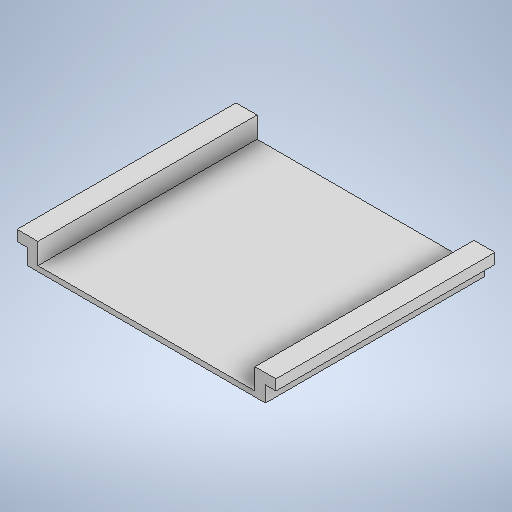
# Autodesk Inventor part: Avionics Cradle (12-13)
Saved by Autodesk Inventor 2025.2 (Build 292293000, 293)
## iProperties
Created: 2025-01-28
Part Number: Avionics Cradle (12-13)
Material: Generic
Document SubType Name: Modeling
Designer: Tia
Density: 1 g/cm^3
Appearance: Default
Author: Tia
Autodesk Inventor part; units mm, degrees
ref_plane "YZ Plane" through (0, 0, 0) normal (1, 0, 0) x (0, 1, 0)
ref_plane "XZ Plane" through (0, 0, 0) normal (0, 1, 0) x (-1, 0, 0)
ref_plane "XY Plane" through (0, 0, 0) normal (0, 0, 1) x (1, 0, 0)
sketch "Sketch2" plane through (0, 0, 0) normal (0, 0, 1) x (1, 0, 0)
  line L0 (-14.9328, -5.3201) -> (-10.9328, -5.3201)
  line L1 (-10.9328, -5.3201) -> (-10.9328, -11.3201)
  line L2 (20.0672, -9.3201) -> (20.0672, -9.3157)
  line L3 (-6.9328, -9.3201) -> (-6.9328, -1.3201)
  line L4 (-6.9328, -1.3201) -> (-14.9328, -1.3201)
  line L5 (-14.9328, -1.3201) -> (-14.9328, -5.3201)
  line L6 (-14.9328, -5.3201) -> (-10.9328, -5.3201)
  line L7 (-14.9328, -1.3201) -> (-6.9328, -1.3201)
  line L8 (-6.9328, -1.3201) -> (-6.9328, -9.3201)
  line L9 (16.0672, -9.3157) -> (16.0672, -9.3201)
  line L10 (-10.9328, -11.3201) -> (-10.9328, -5.3201)
  line L11 (-10.9328, -5.3201) -> (-14.9328, -5.3201)
  line L12 (-14.9328, -1.3201) -> (-14.9328, -5.3201)
  line L13 (-10.9328, -11.3201) -> (34.4422, -11.3201)
  line L14 (-10.9328, -11.3201) -> (34.4422, -11.3201) construction
  line L15 (34.4422, -11.3201) -> (34.4422, -9.3201)
  line L16 (-6.9328, -9.3201) -> (34.4422, -9.3201)
  point P0 (0, 0)
  point P1 (-14.9328, 16.2146)
  point P2 (20.0672, -10.3179)
  point P3 (-12.9328, -5.3201)
  point P4 (-14.9328, -5.3201)
  dimension "d2" = 8
  dimension "d3" = 90
  dimension "d4" = 4
  dimension "d5" = 90
  dimension "d6" = 4
  dimension "d7" = 90
  dimension "d23" = 45.375
  dimension "d24" = 0
  dimension "d25" = 2
  constraints: 34 end point, 8 perpendicular, 4 horizontal, 2 collinear, 2 vertical, 1 midpoint, 1 point on line, 2 other
  measures "d2" distance of L3.end L4.end
  measures "d3" angle of L4 L3
  measures "d4" distance of L4.end L5.end
  measures "d5" angle of L5 L4
  measures "d6" distance of L5.end L6.end
  measures "d7" angle of L6 L5
  measures "d23" distance of L1.end L13.end
  measures "d24" distance between parallel lines of L13 L14
  measures "d25" distance of L13.end L15.end
extrude "Extrusion4" add sketch "Sketch2" along normal blind 83.525
mirror "Mirror4" about plane through (34.4422, -11.3201, 0) normal (1, 0, 0) of "Extrusion4"
body "Solid4"
